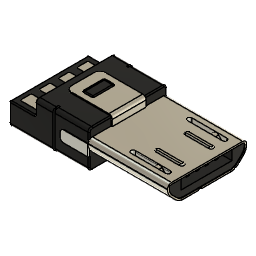
Micro-B (Autodesk Fusion 360 design; units mm, degrees)
Autodesk Fusion 360 part; units mm, degrees
sketch "Sketch1" plane through (0, 0, 0) normal (0, 0, 1) x (1, 0, 0)
  line L0 (3.35, 3.5) -> (-3.35, 3.5)
  line L1 (-3.35, 3.5) -> (-3.35, -3.5)
  line L2 (-3.35, -3.5) -> (3.35, -3.5)
  line L3 (3.35, -3.5) -> (3.35, 3.5)
  line L4 (3.35, 3.5) -> (-3.35, -3.5) construction
  line L5 (-3.35, 3.5) -> (3.35, -3.5) construction
  dimension "d1" = 6.7
  dimension "d2" = 7
  constraint horizontal L0
  constraint perpendicular L0 L1
  constraint parallel L0 L2
  constraint parallel L1 L3
  constraint coincident L4 origin
  constraint coincident L5 origin
  measures "d1" distance of L1.end L2.end
  measures "d2" distance of L0.end L1.end
extrude "Extrude1" add sketch "Sketch1" along normal blind 3.3
sketch "Sketch2" plane through (0, 0, 3.3) normal (0, 0, 1) x (-1, 0, 0)
  line L0 (-3.35, 3.5) -> (-3.35, -3.5)
  line L1 (-3.35, -3.5) -> (3.35, -3.5)
  line L2 (3.35, -3.5) -> (3.35, 3.5)
  line L3 (3.35, 3.5) -> (-3.35, 3.5)
  line L4 (3.35, -3.5) -> (1.35, -3.5)
  line L5 (1.35, -3.5) -> (1.35, 3.5)
  line L6 (1.35, 3.5) -> (3.35, 3.5)
  line L7 (3.35, 3.5) -> (3.35, -3.5)
  dimension "d5" = 2
  constraint horizontal L4
  constraint vertical L5
  constraint horizontal L6
  constraint vertical L7
  constraint coincident L3 L5.end
  constraint coincident L1.end L2.start
  measures "d5" distance of L1.end L4.end
extrude "Extrude2" cut sketch "Sketch2" against normal blind 1.3 contours L1 L2 L3 L4 L5 L6 L7
sketch "Sketch3" plane through (0, 0, 2) normal (0, 0, 1) x (-1, 0, 0)
  line L0 (3.35, 3.5) -> (1.35, 3.5)
  line L1 (1.35, 3.5) -> (1.35, -3.5)
  line L2 (1.35, -3.5) -> (3.35, -3.5)
  line L3 (3.35, -3.5) -> (3.35, 3.5)
  circle A0 centre (2.35, -2.5) radius 0.75
  line L4 (3.2, -3) -> (1.5, -3)
  line L5 (1.5, -3) -> (1.5, -2)
  line L6 (1.5, -2) -> (3.2, -2)
  line L7 (3.2, -2) -> (3.2, -3)
  line L8 (3.2, -3) -> (1.5, -2) construction
  line L9 (1.5, -3) -> (3.2, -2) construction
  line L10 (3.2, -0.35) -> (1.5, -0.35)
  line L11 (1.5, -0.35) -> (1.5, -1.35)
  line L12 (1.5, -1.35) -> (3.2, -1.35)
  line L13 (3.2, -1.35) -> (3.2, -0.35)
  line L14 (3.2, -0.35) -> (1.5, -1.35) construction
  line L15 (1.5, -0.35) -> (3.2, -1.35) construction
  point P0 (2.35, -2.5)
  point P1 (2.35, -0.85)
  dimension "d8" = 1.5
  dimension "d9" = 1
  dimension "d10" = 1
  dimension "d161" = 1.7
  dimension "d162" = 1
  dimension "d165" = 1.7
  dimension "d166" = 1
  dimension "d167" = 1.65
  dimension "d168" = 1
  constraint horizontal L4
  constraint perpendicular L4 L5
  constraint parallel L4 L6
  constraint parallel L5 L7
  constraint coincident L8 P0
  constraint coincident L9 P0
  constraint coincident P0 A0.centre
  constraint horizontal L10
  constraint perpendicular L10 L11
  constraint parallel L10 L12
  constraint parallel L11 L13
  constraint coincident L14 P1
  constraint coincident L15 P1
  measures "d8" diameter of A0
  measures "d9" distance of L2 P0
  measures "d10" distance of L1 P0
  measures "d161" distance of L5.end L6.end
  measures "d162" distance of L4.end L5.end
  measures "d165" distance of L11.end L12.end
  measures "d166" distance of L10.end L11.end
  measures "d167" distance of P0 P1
  measures "d168" distance of L3 P1
extrude "Extrude3" add sketch "Sketch3" along normal blind 0.001 contours A0 L4 L6 | A0 L4 L6 L7 | A0 L4 L5 L6
mirror "Mirror1" about plane through (0, 0, 0) normal (0, 1, 0) of "Extrude3"
sketch "Sketch4" plane through (0, 0, 0) normal (0, 0, -1) x (1, 0, 0)
  line L0 (3.35, -3.5) -> (3.35, 3.5)
  line L1 (3.35, 3.5) -> (-3.35, 3.5)
  line L2 (-3.35, 3.5) -> (-3.35, -3.5)
  line L3 (-3.35, -3.5) -> (3.35, -3.5)
  line L4 (-2.75, 2.75) -> (-1.95, 2.75)
  line L5 (-1.95, 2.75) -> (-1.95, -2.75)
  line L6 (-1.95, -2.75) -> (-2.75, -2.75)
  line L7 (-2.75, -2.75) -> (-2.75, 2.75)
  line L8 (-2.75, 2.75) -> (-1.95, -2.75) construction
  line L9 (-1.95, 2.75) -> (-2.75, -2.75) construction
  line L10 (0.35, -3.5) -> (0.2, -3.5)
  line L11 (0.2, -3.5) -> (0.2, 3.5)
  line L12 (0.2, 3.5) -> (0.35, 3.5)
  line L13 (0.35, 3.5) -> (0.35, -3.5)
  line L14 (3.35, -1.5) -> (-0.65, -1.5)
  line L15 (-0.65, -1.5) -> (-0.65, 1.5)
  line L16 (-0.65, 1.5) -> (3.35, 1.5)
  line L17 (3.35, 1.5) -> (3.35, -1.5)
  line L18 (3.35, -1.5) -> (3.45, -1.5)
  line L19 (3.45, -1.5) -> (3.45, 1.5)
  line L20 (3.45, 1.5) -> (3.35, 1.5)
  line L21 (3.35, 1.5) -> (3.35, -1.5)
  point P0 (-2.35, 0)
  dimension "d15" = 0.8
  dimension "d16" = 5.5
  dimension "d17" = 1
  dimension "d18" = 3.5
  dimension "d21" = 0.15
  dimension "d22" = 7
  dimension "d23" = 3
  dimension "d26" = 4
  dimension "d27" = 3
  dimension "d28" = 2
  dimension "d29" = 0.1
  dimension "d30" = 3
  constraint horizontal L4
  constraint perpendicular L4 L5
  constraint parallel L4 L6
  constraint parallel L5 L7
  constraint coincident L8 P0
  constraint coincident L9 P0
  constraint horizontal L10
  constraint vertical L11
  constraint horizontal L12
  constraint vertical L13
  constraint coincident L3 L10.start
  constraint horizontal L14
  constraint vertical L15
  constraint horizontal L16
  constraint vertical L17
  constraint coincident L0 L14.start
  constraint horizontal L18
  constraint vertical L19
  constraint horizontal L20
  constraint vertical L21
  measures "d15" distance of L5.end L6.end
  measures "d16" distance of L4.end L5.end
  measures "d17" distance of L2 P0
  measures "d18" distance of L3 P0
  measures "d21" distance of L10.start L10.end
  measures "d22" distance of L10.start L12.end
  measures "d23" distance of L0 L13
  measures "d26" distance of L14.start L14.end
  measures "d27" distance of L14.start L16.end
  measures "d28" distance of L3 L14
  measures "d29" distance of L14.start L18.end
  measures "d30" distance of L14.start L16.end
extrude "Extrude4" cut sketch "Sketch4" against normal blind 0.5 contours L4 L5 L6 L7
extrude "Extrude5" cut sketch "Sketch4" against normal blind 0.2 contours L3 L10 L11 L13 L14 | L11 L13 L14 L16 | L1 L11 L12 L13 L16
extrude "Extrude6" add sketch "Sketch4" along normal blind 0.1 contours L0 L13 L14 L16 L17 L21 | L0 L17 L18 L19 L20 L21 | L11 L13 L14 L16 | L11 L14 L15 L16
extrude "Extrude7" add 1 faces at (3.3833, -0.5, 0) along direction (0, 0, 1) blind 0.75
sketch "Sketch5" plane through (0, 0, -0.1) normal (0, 0, -1) x (1, 0, 0)
  line L0 (-0.65, -1.5) -> (3.45, -1.5)
  line L1 (3.45, -1.5) -> (3.45, 1.5)
  line L2 (3.45, 1.5) -> (-0.65, 1.5)
  line L3 (-0.65, 1.5) -> (-0.65, -1.5)
  line L4 (0.25, 1) -> (1.25, 1)
  line L5 (1.25, 1) -> (1.25, -1)
  line L6 (1.25, -1) -> (0.25, -1)
  line L7 (0.25, -1) -> (0.25, 1)
  line L8 (0.25, 1) -> (1.25, -1) construction
  line L9 (1.25, 1) -> (0.25, -1) construction
  point P0 (0.75, 0)
  dimension "d35" = 1
  dimension "d36" = 2
  dimension "d37" = 1.5
  dimension "d38" = 1.4
  constraint horizontal L4
  constraint perpendicular L4 L5
  constraint parallel L4 L6
  constraint parallel L5 L7
  constraint coincident L8 P0
  constraint coincident L9 P0
  measures "d35" distance of L5.end L6.end
  measures "d36" distance of L4.end L5.end
  measures "d37" distance of L0 P0
  measures "d38" distance of L3 P0
extrude "Extrude8" cut sketch "Sketch5" against normal blind 0.08 contours L4 L5 L6 L7
fillet "Fillet1" radius 0.5 2 edges at (-0.65, -1.5, -0.05) (-0.65, 1.5, -0.05)
fillet "Fillet1" radius 0.15 4 edges at (0.25, 1, -0.06) (1.25, 1, -0.06) (1.25, -1, -0.06) (0.25, -1, -0.06)
fillet "Fillet1" radius 0.3 1 edges at (3.45, 0, -0.1)
sketch "Sketch6" plane through (0, 0, -0.02) normal (0, 0, -1) x (1, 0, 0)
  arc A0 (0.4, 1) -> (0.25, 0.85) centre (0.4, 0.85) ccw
  line L0 (0.25, 0.85) -> (0.25, -0.85)
  arc A1 (0.25, -0.85) -> (0.4, -1) centre (0.4, -0.85) ccw
  line L1 (0.4, -1) -> (1.1, -1)
  arc A2 (1.1, -1) -> (1.25, -0.85) centre (1.1, -0.85) ccw
  line L2 (1.25, -0.85) -> (1.25, 0.85)
  arc A3 (1.25, 0.85) -> (1.1, 1) centre (1.1, 0.85) ccw
  line L3 (1.1, 1) -> (0.4, 1)
  line L4 (1.2, -0.85) -> (1.2, 0.85)
  arc A4 (1.2, 0.85) -> (1.1, 0.95) centre (1.1, 0.85) ccw
  line L5 (1.1, 0.95) -> (0.4, 0.95)
  arc A5 (0.4, 0.95) -> (0.3, 0.85) centre (0.4, 0.85) ccw
  line L6 (0.3, 0.85) -> (0.3, -0.85)
  arc A6 (0.3, -0.85) -> (0.4, -0.95) centre (0.4, -0.85) ccw
  line L7 (0.4, -0.95) -> (1.1, -0.95)
  arc A7 (1.1, -0.95) -> (1.2, -0.85) centre (1.1, -0.85) ccw
  dimension "d47" = -0.05
extrude "Extrude9" add sketch "Sketch6" along normal blind 0.1 contours L4 A4 L5 A5 L6 A6 L7 A7
fillet "Fillet2" radius 0.1 8 edges at (0.75, -0.95, -0.12) (0.3293, -0.9207, -0.12) (0.3, 0, -0.12) (0.3293, 0.9207, -0.12) (0.75, 0.95, -0.12) (1.1707, 0.9207, -0.12) (1.2, 0, -0.12) (1.1707, -0.9207, -0.12)
ref_plane "WorkPlane1" through (1.85, -2.5, 1.65) normal (0, 0, -1) x (-1, 0, 0)
mirror "Mirror2" about plane through (1.85, -2.5, 1.65) normal (0, 0, -1) of "Extrude6", "Extrude7", "Extrude8", "Fillet1", "Extrude9", "Fillet2"
sketch "Sketch7" plane through (0, -3.5, 0) normal (0, -1, 0) x (1, 0, 0)
  line L0 (0.2, 0) -> (0.2, 0.2)
  line L1 (0.2, 0.2) -> (0.35, 0.2)
  line L2 (0.35, 0.2) -> (0.35, 0)
  line L3 (0.35, 0) -> (3.35, 0)
  line L4 (3.35, 0) -> (3.35, 3.3)
  line L5 (3.35, 3.3) -> (-1.35, 3.3)
  line L6 (-1.35, 3.3) -> (-1.35, 2)
  line L7 (-1.35, 2) -> (-3.35, 2)
  line L8 (-3.35, 2) -> (-3.35, 0)
  line L9 (-3.35, 0) -> (0.2, 0)
  line L10 (0.35, 0.2) -> (0.2, 0.2)
  line L11 (0.2, 0.2) -> (0.2, 3.3)
  line L12 (0.2, 3.3) -> (0.35, 3.3)
  line L13 (0.35, 3.3) -> (0.35, 0.2)
  dimension "d54" = 0.15
  constraint horizontal L10
  constraint vertical L11
  constraint horizontal L12
  constraint vertical L13
  constraint coincident L5 L11.end
  constraint coincident L1.end L2.start
  measures "d54" distance of L1.end L0.end
extrude "Extrude10" cut sketch "Sketch7" against normal blind 0.2 contours L1 L5 L10 L11 L12 L13
mirror "Mirror3" about plane through (0, 0, 0) normal (0, 1, 0) of "Extrude10"
sketch "Sketch8" plane through (3.35, 0, 0) normal (1, 0, 0) x (0, 1, 0)
  line L0 (-1.5, 2.55) -> (-1.5, 3.3)
  line L1 (-1.5, 3.3) -> (-3.5, 3.3)
  line L2 (-3.5, 3.3) -> (-3.5, 0)
  line L3 (-3.5, 0) -> (-1.5, 0)
  line L4 (-1.5, 0) -> (-1.5, 0.75)
  line L5 (-1.5, 0.75) -> (1.5, 0.75)
  line L6 (1.5, 0.75) -> (1.5, 0)
  line L7 (1.5, 0) -> (3.5, 0)
  line L8 (3.5, 0) -> (3.5, 3.3)
  line L9 (3.5, 3.3) -> (1.5, 3.3)
  line L10 (1.5, 3.3) -> (1.5, 2.55)
  line L11 (1.5, 2.55) -> (-1.5, 2.55)
  line L12 (1.5, 2.55) -> (3.5, 2.55)
  line L13 (3.5, 2.55) -> (-3.5, 2.55)
  line L14 (-3.5, 2.55) -> (-3.5, 0.75)
  line L15 (-3.5, 0.75) -> (3.5, 0.75)
  line L16 (3.5, 0.75) -> (3.5, 2.55)
  dimension "d59" = 1.8
  constraint coincident L10.end L11.start
  constraint coincident L8 L12.end
  constraint perpendicular L8 L12
  constraint horizontal L13
  constraint vertical L14
  constraint horizontal L15
  constraint vertical L16
  constraint coincident L2 L14.end
  measures "d59" distance of L12.end L15.end
extrude "Extrude11" add sketch "Sketch8" along normal blind 7 contours L2 L5 L8 L11 L12 L13 L14 L15 L16
extrude "Extrude12" add 1 faces at (-3.35, 1.1667, 0.6667) along direction (-1, 0, 0) blind 0.3
sketch "Sketch9" plane through (0, -3.5, 0) normal (0, -1, 0) x (1, 0, 0)
  line L0 (0.35, 3.3) -> (0.35, 0)
  line L1 (0.35, 0) -> (3.35, 0)
  line L2 (3.35, 0) -> (3.35, 0.75)
  line L3 (3.35, 0.75) -> (10.35, 0.75)
  line L4 (10.35, 0.75) -> (10.35, 2.55)
  line L5 (10.35, 2.55) -> (3.35, 2.55)
  line L6 (3.35, 2.55) -> (3.35, 3.3)
  line L7 (3.35, 3.3) -> (0.35, 3.3)
  line L8 (3.35, 2.55) -> (3.35, 0.75)
  line L9 (3.35, 2.15) -> (0.85, 2.15)
  line L10 (0.85, 2.15) -> (0.85, 1.15)
  line L11 (0.85, 1.15) -> (3.35, 1.15)
  line L12 (3.35, 1.15) -> (3.35, 2.15)
  dimension "d64" = 2.5
  dimension "d65" = 1
  dimension "d66" = 1.15
  constraint coincident L5.end L6.start
  constraint coincident L2.end L3.start
  constraint horizontal L9
  constraint vertical L10
  constraint horizontal L11
  constraint vertical L12
  constraint coincident L8 L9.start
  measures "d64" distance of L9.start L9.end
  measures "d65" distance of L9.start L11.end
  measures "d66" distance of L7 L9
extrude "Extrude13" cut sketch "Sketch9" against normal blind 0.05 contours L0 L1 L2 L6 L7 L8 L9 L10 L11
fillet "Fillet3" radius 0.3 2 edges at (0.85, -3.475, 2.15) (0.85, -3.475, 1.15)
mirror "Mirror4" about plane through (0, 0, 0) normal (0, 1, 0) of "Extrude13", "Fillet3"
sketch "Sketch10" plane through (0, 0, 2.55) normal (0, 0, 1) x (-1, 0, 0)
  line L0 (-3.35, -1.5) -> (-3.45, -1.5)
  line L1 (-3.45, -1.5) -> (-3.45, 1.5)
  line L2 (-3.45, 1.5) -> (-3.35, 1.5)
  line L3 (-3.35, 1.5) -> (-3.35, 3.45)
  line L4 (-3.35, 3.45) -> (-3.35, 3.5)
  line L5 (-3.35, 3.5) -> (-10.35, 3.5)
  line L6 (-10.35, 3.5) -> (-10.35, -3.5)
  line L7 (-10.35, -3.5) -> (-3.35, -3.5)
  line L8 (-3.35, -3.5) -> (-3.35, -3.45)
  line L9 (-3.35, -3.45) -> (-3.35, -1.5)
  line L10 (-6.1, -2.3) -> (-9.6, -2.3)
  line L11 (-9.6, -2.3) -> (-9.6, -2.7)
  line L12 (-9.6, -2.7) -> (-6.1, -2.7)
  line L13 (-6.1, -2.7) -> (-6.1, -2.3)
  line L14 (-6.1, -2.3) -> (-9.6, -2.7) construction
  line L15 (-9.6, -2.3) -> (-6.1, -2.7) construction
  line L16 (-7.1, -1.1) -> (-9.6, -1.1)
  line L17 (-9.6, -1.1) -> (-9.6, -1.5)
  line L18 (-9.6, -1.5) -> (-7.1, -1.5)
  line L19 (-7.1, -1.5) -> (-7.1, -1.1)
  line L20 (-7.1, -1.1) -> (-9.6, -1.5) construction
  line L21 (-9.6, -1.1) -> (-7.1, -1.5) construction
  point P0 (-7.85, -2.5)
  point P1 (-8.35, -1.3)
  dimension "d73" = 0.4
  dimension "d74" = 3.5
  dimension "d75" = 2.5
  dimension "d76" = 1
  dimension "d77" = 2.5
  dimension "d78" = 0.4
  dimension "d79" = 1
  dimension "d80" = 2
  constraint horizontal L10
  constraint perpendicular L10 L11
  constraint parallel L10 L12
  constraint parallel L11 L13
  constraint coincident L14 P0
  constraint coincident L15 P0
  constraint horizontal L16
  constraint perpendicular L16 L17
  constraint parallel L16 L18
  constraint parallel L17 L19
  constraint coincident L20 P1
  constraint coincident L21 P1
  measures "d73" distance of L10.end L11.end
  measures "d74" distance of L11.end L12.end
  measures "d75" distance of L6 P0
  measures "d76" distance of L7 P0
  measures "d77" distance of L17.end L18.end
  measures "d78" distance of L16.end L17.end
  measures "d79" distance of L10 P1
  measures "d80" distance of L6 P1
extrude "Extrude14" cut sketch "Sketch10" against normal blind 0.5 contours L10 L11 L12 L13
extrude "Extrude15" add sketch "Sketch10" along normal blind 0.1 contours L16 L17 L18 L19
sketch "Sketch11" plane through (0, 0, 2.05) normal (0, 0, 1) x (-1, 0, 0)
  line L0 (-6.1, -2.7) -> (-6.1, -2.3)
  line L1 (-6.1, -2.3) -> (-9.6, -2.3)
  line L2 (-9.6, -2.3) -> (-9.6, -2.7)
  line L3 (-9.6, -2.7) -> (-6.1, -2.7)
  line L4 (-6.125, -2.325) -> (-9.575, -2.325)
  line L5 (-9.575, -2.325) -> (-9.575, -2.675)
  line L6 (-9.575, -2.675) -> (-6.125, -2.675)
  line L7 (-6.125, -2.675) -> (-6.125, -2.325)
  line L8 (-8.075, -2.675) -> (-9.075, -2.675)
  line L9 (-9.075, -2.675) -> (-9.075, -2.325)
  line L10 (-9.075, -2.325) -> (-8.075, -2.325)
  line L11 (-8.075, -2.325) -> (-8.075, -2.675)
  dimension "d85" = -0.025
  dimension "d86" = 1
  dimension "d87" = 0.5
  dimension "d88" = 0.35
  constraint horizontal L8
  constraint vertical L9
  constraint horizontal L10
  constraint vertical L11
  constraint coincident L6 L8.start
  measures "d86" distance of L8.start L8.end
  measures "d87" distance of L5 L9
  measures "d88" distance of L8.end L9.end
extrude "Extrude16" add sketch "Sketch11" along normal blind 0.5 contours L4 L6 L8 L9 L10 L11
chamfer "Chamfer1" distance 0.5 distance2 0.5 1 edges at (9.075, 2.5, 2.55) measured on face at (8.7417, 2.4417, 2.55)
chamfer "Chamfer1" distance 0.2 distance2 0.5 1 edges at (8.075, 2.5, 2.55) measured on face at (8.7417, 2.4417, 2.55)
fillet "Fillet4" radius 0.3 2 edges at (8.575, 2.5, 2.55) (8.275, 2.5, 2.55)
fillet "Fillet4" radius 0.2 8 edges at (9.6, 2.7, 2.3) (9.6, 2.3, 2.3) (6.1, 2.3, 2.3) (6.1, 2.7, 2.3) (7.1, 1.1, 2.6) (7.1, 1.5, 2.6) (9.6, 1.1, 2.6) (9.6, 1.5, 2.6)
fillet "Fillet5" radius 0.1 4 edges at (7.1, 1.3, 2.65) (8.35, 1.1, 2.65) (9.6, 1.3, 2.65) (8.35, 1.5, 2.65)
mirror "Mirror5" about plane through (0, 0, 0) normal (0, 1, 0) of "Extrude14", "Extrude15", "Extrude16", "Chamfer1", "Fillet4", "Fillet5"
sketch "Sketch12" plane through (0, 0, 0.75) normal (0, 0, -1) x (1, 0, 0)
  line L0 (3.45, -1.5) -> (3.35, -1.5)
  line L1 (3.35, -1.5) -> (3.35, -3.45)
  line L2 (3.35, -3.45) -> (3.35, -3.5)
  line L3 (3.35, -3.5) -> (10.35, -3.5)
  line L4 (10.35, -3.5) -> (10.35, 3.5)
  line L5 (10.35, 3.5) -> (3.35, 3.5)
  line L6 (3.35, 3.5) -> (3.35, 3.45)
  line L7 (3.35, 3.45) -> (3.35, 1.5)
  line L8 (3.35, 1.5) -> (3.45, 1.5)
  line L9 (3.45, 1.5) -> (3.45, -1.5)
  arc A0 (6.0406, -0.465) -> (6.3156, -0.74) centre (6.3156, -0.465) ccw
  arc A1 (6.2406, -0.465) -> (6.22, -0.3765) centre (6.0406, -0.465) ccw
  arc A2 (4.8906, -0.465) -> (5.1656, -0.74) centre (5.1656, -0.465) ccw
  line L10 (6.0406, -0.465) -> (6.0406, -0.515)
  arc A3 (5.7656, -0.24) -> (5.4906, -0.515) centre (5.7656, -0.515) ccw
  arc A4 (11.2406, -0.465) -> (11.22, -0.3765) centre (11.0406, -0.465) ccw
  arc A5 (10.2156, -0.74) -> (10.4906, -0.465) centre (10.2156, -0.465) ccw
  arc A6 (6.2406, -0.465) -> (6.3156, -0.54) centre (6.3156, -0.465) ccw
  arc A7 (10.3112, -0.3765) -> (10.2906, -0.465) centre (10.4906, -0.465) ccw
  arc A8 (5.2156, -0.54) -> (5.2906, -0.465) centre (5.2156, -0.465) ccw
  arc A9 (6.3656, -0.74) -> (6.6406, -0.465) centre (6.3656, -0.465) ccw
  line L11 (6.3656, -0.54) -> (6.3156, -0.54)
  arc A10 (5.0906, -0.465) -> (5.1656, -0.54) centre (5.1656, -0.465) ccw
  line L12 (5.1656, -0.54) -> (5.2156, -0.54)
  line L13 (6.3656, -0.74) -> (6.3156, -0.74)
  line L14 (11.3656, -0.74) -> (11.3156, -0.74)
  line L15 (6.3656, -0.74) -> (6.3156, -0.74)
  line L16 (5.4906, -0.465) -> (5.4906, -0.515)
  arc A11 (6.3656, -0.74) -> (6.6406, -0.465) centre (6.3656, -0.465) ccw
  arc A12 (11.2406, -0.465) -> (11.3156, -0.54) centre (11.3156, -0.465) ccw
  arc A13 (8.8656, -0.54) -> (8.9406, -0.465) centre (8.8656, -0.465) ccw
  line L17 (6.3656, -0.54) -> (6.3156, -0.54)
  line L18 (11.0406, -0.515) -> (11.0406, -0.465)
  arc A14 (6.3656, -0.54) -> (6.4406, -0.465) centre (6.3656, -0.465) ccw
  arc A15 (6.2406, -0.465) -> (6.3156, -0.54) centre (6.3156, -0.465) ccw
  line L19 (7.6656, -0.54) -> (7.7156, -0.54)
  arc A16 (11.0406, -0.465) -> (11.3156, -0.74) centre (11.3156, -0.465) ccw
  line L20 (10.4906, -0.515) -> (10.4906, -0.465)
  arc A17 (6.0406, -0.515) -> (5.7656, -0.24) centre (5.7656, -0.515) ccw
  arc A18 (11.3656, -0.74) -> (11.6406, -0.465) centre (11.3656, -0.465) ccw
  arc A19 (5.3112, -0.3765) -> (5.2906, -0.465) centre (5.4906, -0.465) ccw
  arc A20 (10.0906, -0.465) -> (10.1656, -0.54) centre (10.1656, -0.465) ccw
  arc A21 (5.2156, -0.74) -> (5.4906, -0.465) centre (5.2156, -0.465) ccw
  arc A22 (4.8906, -0.465) -> (5.1656, -0.74) centre (5.1656, -0.465) ccw
  arc A23 (11.0406, -0.515) -> (10.7656, -0.24) centre (10.7656, -0.515) ccw
  arc A24 (6.0406, -0.465) -> (6.3156, -0.74) centre (6.3156, -0.465) ccw
  arc A25 (9.8906, -0.465) -> (10.1656, -0.74) centre (10.1656, -0.465) ccw
  arc A26 (5.0906, -0.465) -> (5.1656, -0.54) centre (5.1656, -0.465) ccw
  arc A27 (6.0406, -0.515) -> (5.7656, -0.24) centre (5.7656, -0.515) ccw
  arc A28 (6.2406, -0.465) -> (6.22, -0.3765) centre (6.0406, -0.465) ccw
  arc A29 (5.3112, -0.3765) -> (5.2906, -0.465) centre (5.4906, -0.465) ccw
  arc A30 (5.2156, -0.74) -> (5.4906, -0.465) centre (5.2156, -0.465) ccw
  arc A31 (5.7656, -0.24) -> (5.4906, -0.515) centre (5.7656, -0.515) ccw
  arc A32 (5.2156, -0.54) -> (5.2906, -0.465) centre (5.2156, -0.465) ccw
  line L21 (3.7906, 3.8194) -> (3.7906, -2.5806)
  line L22 (12.1906, 3.8194) -> (3.7906, 3.8194)
  line L23 (3.7906, -2.5806) -> (12.1906, -2.5806)
  line L24 (8.5406, -0.465) -> (8.5406, -0.515)
  line L25 (9.1406, 0.51) -> (9.1406, -0.465)
  line L26 (10.0906, 0.51) -> (10.0906, -0.465)
  line L27 (11.4406, 0.51) -> (11.4406, -0.465)
  arc A33 (5.7656, -0.04) -> (5.3112, -0.3765) centre (5.7656, -0.515) ccw
  line L28 (9.8906, 0.51) -> (9.8906, -0.465)
  line L29 (11.1, -2.515) -> (11.1, 3.735)
  arc A34 (8.2656, -0.24) -> (7.9906, -0.515) centre (8.2656, -0.515) ccw
  line L30 (4.45, 0.61) -> (11.1, 0.61)
  line L31 (12.1906, -2.5806) -> (12.1906, 3.8194)
  line L32 (4.45, -2.515) -> (11.1, -2.515)
  line L33 (11.1, 0.61) -> (12.1906, 0.61)
  line L34 (11.1, 0.71) -> (12.1906, 0.71)
  line L35 (4.45, 0.71) -> (11.1, 0.71)
  circle A35 centre (9.1906, 2.6194) radius 0.3732
  line L36 (11.6406, 0.51) -> (12.1906, 0.51)
  line L37 (11.4406, 0.51) -> (11.4406, 0.71)
  line L38 (8.9406, 0.51) -> (8.9406, 0.71)
  arc A36 (7.7156, -0.54) -> (7.7906, -0.465) centre (7.7156, -0.465) ccw
  line L39 (5.0906, 0.51) -> (5.0906, 0.71)
  line L40 (6.6406, 0.51) -> (6.6406, -0.465)
  line L41 (5.0906, 0.51) -> (5.0906, -0.465)
  arc A37 (8.72, -0.3765) -> (8.2656, -0.04) centre (8.2656, -0.515) ccw
  line L42 (4.45, 0.51) -> (3.7906, 0.51)
  arc A38 (7.8112, -0.3765) -> (7.7906, -0.465) centre (7.9906, -0.465) ccw
  line L43 (4.45, 0.71) -> (3.7906, 0.71)
  line L44 (8.9406, 0.51) -> (8.9406, -0.465)
  line L45 (7.5906, 0.51) -> (7.5906, 0.71)
  line L46 (4.45, 0.51) -> (11.1, 0.51)
  line L47 (10.0906, 0.51) -> (10.0906, 0.71)
  line L48 (6.4406, 0.51) -> (6.4406, 0.71)
  line L49 (7.6656, -0.74) -> (7.7156, -0.74)
  line L50 (6.6406, 0.51) -> (6.6406, -0.465)
  arc A39 (6.22, -0.3765) -> (5.7656, -0.04) centre (5.7656, -0.515) ccw
  arc A40 (8.5406, -0.465) -> (8.8156, -0.74) centre (8.8156, -0.465) ccw
  line L51 (7.5906, 0.51) -> (7.5906, -0.465)
  line L52 (4.8906, 0.51) -> (4.8906, -0.465)
  arc A41 (8.7406, -0.465) -> (8.8156, -0.54) centre (8.8156, -0.465) ccw
  line L53 (4.45, 3.735) -> (4.45, -2.515)
  arc A42 (8.5406, -0.515) -> (8.2656, -0.24) centre (8.2656, -0.515) ccw
  line L54 (10.1656, -0.74) -> (10.2156, -0.74)
  arc A43 (8.8656, -0.74) -> (9.1406, -0.465) centre (8.8656, -0.465) ccw
  line L55 (11.3656, -0.54) -> (11.3156, -0.54)
  line L56 (5.1656, -0.74) -> (5.2156, -0.74)
  line L57 (6.4406, 0.51) -> (6.4406, -0.465)
  arc A44 (8.7406, -0.465) -> (8.72, -0.3765) centre (8.5406, -0.465) ccw
  line L58 (7.9906, -0.515) -> (7.9906, -0.465)
  arc A45 (7.5906, -0.465) -> (7.6656, -0.54) centre (7.6656, -0.465) ccw
  arc A46 (5.7656, -0.04) -> (5.3112, -0.3765) centre (5.7656, -0.515) ccw
  arc A47 (11.22, -0.3765) -> (10.7656, -0.04) centre (10.7656, -0.515) ccw
  arc A48 (10.7656, -0.04) -> (10.3112, -0.3765) centre (10.7656, -0.515) ccw
  arc A49 (10.2156, -0.54) -> (10.2906, -0.465) centre (10.2156, -0.465) ccw
  arc A50 (8.2656, -0.04) -> (7.8112, -0.3765) centre (8.2656, -0.515) ccw
  arc A51 (11.3656, -0.54) -> (11.4406, -0.465) centre (11.3656, -0.465) ccw
  arc A52 (7.7156, -0.74) -> (7.9906, -0.465) centre (7.7156, -0.465) ccw
  line L59 (7.3906, 0.51) -> (7.3906, -0.465)
  line L60 (8.8656, -0.54) -> (8.8156, -0.54)
  line L61 (11.6406, 0.51) -> (11.6406, -0.465)
  arc A53 (10.7656, -0.24) -> (10.4906, -0.515) centre (10.7656, -0.515) ccw
  line L62 (10.1656, -0.54) -> (10.2156, -0.54)
  line L63 (8.8656, -0.74) -> (8.8156, -0.74)
  arc A54 (7.3906, -0.465) -> (7.6656, -0.74) centre (7.6656, -0.465) ccw
  circle A55 centre (9.1906, -1.3806) radius 0.3732
  line L64 (3.7906, 0.71) -> (3.45, 0.71)
  line L65 (3.7906, 0.51) -> (3.45, 0.51)
  point P0 (6.6406, -0.74)
  point P1 (4.8906, -0.74)
  point P2 (6.0406, -0.74)
  point P3 (5.4906, -0.24)
  point P4 (6.0406, -0.24)
  point P5 (5.4906, -0.74)
  dimension "d103" = 0.2
  dimension "d104" = 0.1
  dimension "d105" = 0.1
  dimension "d106" = 1.25
  dimension "d107" = 1.25
  dimension "d108" = 0.6
  dimension "d109" = 1.75
  dimension "d110" = 0.6
  dimension "d111" = 0.5
  dimension "d112" = 0.5
  dimension "d113" = 0.275
  dimension "d114" = 0.275
  dimension "d115" = 0.275
  dimension "d116" = 0.275
  dimension "d117" = 1.75
  dimension "d118" = 0.275
  dimension "d119" = 0.275
  dimension "d120" = 1.75
  dimension "d121" = 0.275
  dimension "d122" = 0.275
  constraint midpoint L30.start L53
  constraint perpendicular L30 L53
  constraint coincident L42.start L53
  constraint coincident L46.end L29
  constraint perpendicular L29 L46
  constraint coincident L35.start L53
  constraint coincident L34.start L29
  constraint perpendicular L29 L35
  constraint coincident L40.start L46
  constraint perpendicular L46 L50
  constraint coincident L52.start L46
  constraint perpendicular L46 L52
  constraint perpendicular L13 L50
  constraint perpendicular L52 L56
  constraint perpendicular L10 L13
  constraint perpendicular L16 L56
  constraint coincident P0 L50
  constraint coincident P0 L13
  constraint tangent A9 L50
  constraint tangent A9 L13
  constraint coincident P2 L13
  constraint coincident P2 L10
  constraint tangent L13 A24
  constraint tangent L10 A24
  constraint equal A9 A24
  constraint coincident P5 L56
  constraint coincident P5 L16
  constraint tangent A30 L56
  constraint tangent L16 A30
  constraint equal A9 A30
  constraint coincident P1 L52
  constraint coincident P1 L56
  constraint tangent A22 L52
  constraint tangent A22 L56
  constraint equal A9 A22
  constraint coincident P4 L10
  constraint tangent L10 A27
  constraint coincident P3 L16
  constraint tangent A3 L16
  constraint equal A3 A27
  constraint coincident A3.start A17.end
  constraint coincident L39.end L35
  constraint perpendicular L35 L39
  constraint coincident L48.end L35
  constraint perpendicular L35 L48
  constraint perpendicular L15 L40
  constraint tangent A11 L40
  constraint tangent L15 A11
  constraint tangent A0 L15
  constraint equal A0 A11
  constraint equal A11 A21
  constraint equal A2 A11
  constraint equal A17 A31
  constraint perpendicular L49 L59
  constraint tangent L25 A43
  constraint tangent L49 A52
  constraint equal A43 A52
  constraint tangent A40 L63
  constraint perpendicular L28 L54
  constraint tangent A18 L61
  constraint tangent A5 L54
  constraint equal A5 A18
  constraint tangent L14 A16
  constraint coincident A43.start L63
  constraint tangent L24 A42
  constraint tangent L58 A52
  constraint coincident A4.centre L18.end
  constraint tangent L18 A16
  constraint coincident A5.end A7.centre
  constraint tangent A5 L20
  constraint coincident L45.end L35
  constraint perpendicular L35 L45
  constraint coincident L38.end L35
  constraint perpendicular L35 L38
  constraint coincident L47.end L35
  constraint perpendicular L35 L47
  constraint coincident L33.end L31
  constraint perpendicular L31 L33
  constraint coincident L36.end L31
  constraint perpendicular L31 L36
  constraint coincident L34.end L31
  constraint perpendicular L31 L34
  constraint coincident L37.end L34
  constraint perpendicular L34 L37
  constraint coincident L42.end L21
  constraint perpendicular L21 L42
  constraint coincident L43.end L21
  constraint perpendicular L21 L43
  constraint coincident L9 L64.end
  constraint perpendicular L9 L64
  constraint coincident L9 L65.end
  constraint perpendicular L9 L65
  measures "d104" distance of L30 L46
  measures "d105" distance of L30 L35
  measures "d106" distance of L40.start P0
  measures "d107" distance of P1 L52.start
  measures "d108" distance of P0 P2
  measures "d109" distance of L50 L52
  measures "d110" distance of P1 P5
  measures "d111" distance of P2 P4
  measures "d112" distance of P3 P5
  measures "d113" radius of A9
  measures "d114" radius of A27
  measures "d115" radius of A11
  measures "d116" radius of A17
  measures "d117" distance of L25 L59
  measures "d118" radius of A43
  measures "d119" radius of A42
  measures "d120" distance of L28 L61
  measures "d121" radius of A18
  measures "d122" radius of A23
extrude "Extrude17" cut sketch "Sketch12" against normal blind 0.1 contours L9 L21 L64 L65 | L21 L42 L43 L53 | L30 L39 L46 L53 | L30 L35 L39 L53 | A0 A1 A2 L10 A3 A6 A8 A9 L11 A10 L12 L13 L15 L16 A11 L17 A14 A15 A17 A19 A21 A22 A24 A26 A27 A28 A29 A30 A31 A32 A33 L40 L41 L46 L50 A39 L52 L56 L57 A46 | L30 L35 L45 L48 | L30 L45 L46 L48 | L4 L30 L35 L47 | L4 L30 L46 L47 | L30 L35 L38 L47 | A13 L19 L24 L25 A34 A36 A37 A38 L44 L46 L49 A40 L51 A41 A42 A43 A44 L58 A45 A50 A52 L59 L60 L63 A54 | L30 L38 L46 L47
fillet "Fillet6" radius 0.1 8 edges at (8.9406, -0.71, 0.8) (9.1406, -0.51, 0.8) (7.5906, -0.71, 0.8) (7.3906, -0.51, 0.8) (6.6406, -0.51, 0.8) (6.4406, -0.71, 0.8) (5.0906, -0.71, 0.8) (4.8906, -0.51, 0.8)
chamfer "Chamfer2" distance 1 distance2 1 2 edges at (6.85, -3.5, 0.75) (6.85, 3.5, 0.75) measured on face at (8.0167, -3.5, 1.8167) measured on face at (6.7016, 2.5791, 0.75)
fillet "Fillet7" radius 0.35 2 edges at (6.85, -3.5, 2.55) (6.85, 3.5, 2.55)
fillet "Fillet7" radius 1 4 edges at (6.85, -3.5, 1.75) (6.85, -2.5, 0.75) (6.85, 2.5, 0.75) (6.85, 3.5, 1.75)
sketch "Sketch13" plane through (10.35, 0, 0) normal (1, 0, 0) x (0, 1, 0)
  arc A0 (3.2071, 1.4571) -> (3.5, 2.1642) centre (2.5, 2.1642) ccw
  line L0 (3.5, 2.1642) -> (3.5, 2.2)
  arc A1 (3.5, 2.2) -> (3.15, 2.55) centre (3.15, 2.2) ccw
  line L1 (3.15, 2.55) -> (-3.15, 2.55)
  arc A2 (-3.15, 2.55) -> (-3.5, 2.2) centre (-3.15, 2.2) ccw
  line L2 (-3.5, 2.2) -> (-3.5, 2.1642)
  arc A3 (-3.5, 2.1642) -> (-3.2071, 1.4571) centre (-2.5, 2.1642) ccw
  line L3 (-3.2071, 1.4571) -> (-2.7929, 1.0429)
  arc A4 (-2.7929, 1.0429) -> (-2.0858, 0.75) centre (-2.0858, 1.75) ccw
  line L4 (-2.0858, 0.75) -> (-0.71, 0.75)
  line L5 (-0.71, 0.75) -> (-0.71, 0.85)
  line L6 (-0.71, 0.85) -> (-0.51, 0.85)
  line L7 (-0.51, 0.85) -> (-0.51, 0.75)
  line L8 (-0.51, 0.75) -> (2.0858, 0.75)
  arc A5 (2.0858, 0.75) -> (2.7929, 1.0429) centre (2.0858, 1.75) ccw
  line L9 (2.7929, 1.0429) -> (3.2071, 1.4571)
  line L10 (-0.71, 0.75) -> (-0.51, 0.75)
  line L11 (2.6868, 1.149) -> (3.101, 1.5632)
  arc A6 (3.101, 1.5632) -> (3.35, 2.1642) centre (2.5, 2.1642) ccw
  line L12 (3.35, 2.1642) -> (3.35, 2.2)
  arc A7 (3.35, 2.2) -> (3.15, 2.4) centre (3.15, 2.2) ccw
  line L13 (3.15, 2.4) -> (-3.15, 2.4)
  arc A8 (-3.15, 2.4) -> (-3.35, 2.2) centre (-3.15, 2.2) ccw
  line L14 (-3.35, 2.2) -> (-3.35, 2.1642)
  arc A9 (-3.35, 2.1642) -> (-3.101, 1.5632) centre (-2.5, 2.1642) ccw
  line L15 (-3.101, 1.5632) -> (-2.6868, 1.149)
  arc A10 (-2.6868, 1.149) -> (-2.0858, 0.9) centre (-2.0858, 1.75) ccw
  line L16 (-2.0858, 0.9) -> (-0.86, 0.9)
  line L17 (-0.86, 0.9) -> (-0.86, 1)
  line L18 (-0.86, 1) -> (-0.36, 1)
  line L19 (-0.36, 1) -> (-0.36, 0.9)
  line L20 (-0.36, 0.9) -> (2.0858, 0.9)
  arc A11 (2.0858, 0.9) -> (2.6868, 1.149) centre (2.0858, 1.75) ccw
  line L21 (-0.86, 0.9) -> (-0.36, 0.9)
  dimension "d133" = -0.15
  constraint coincident L4.end L5.start
  constraint coincident L7.end L8.start
extrude "Extrude18" cut sketch "Sketch13" against normal blind 0.05 contours L11 A6 L12 A7 L13 A8 L14 A9 L15 A10 L16 L17 L18 L19 L20 A11 | L17 L18 L19 L21
sketch "Sketch14" plane through (10.3, 0, 0) normal (1, 0, 0) x (0, 1, 0)
  line L0 (-2.0858, 0.9) -> (2.0858, 0.9)
  arc A0 (2.0858, 0.9) -> (2.6868, 1.149) centre (2.0858, 1.75) ccw
  line L1 (2.6868, 1.149) -> (3.101, 1.5632)
  arc A1 (3.101, 1.5632) -> (3.35, 2.1642) centre (2.5, 2.1642) ccw
  line L2 (3.35, 2.1642) -> (3.35, 2.2)
  arc A2 (3.35, 2.2) -> (3.15, 2.4) centre (3.15, 2.2) ccw
  line L3 (3.15, 2.4) -> (-3.15, 2.4)
  arc A3 (-3.15, 2.4) -> (-3.35, 2.2) centre (-3.15, 2.2) ccw
  line L4 (-3.35, 2.2) -> (-3.35, 2.1642)
  arc A4 (-3.35, 2.1642) -> (-3.101, 1.5632) centre (-2.5, 2.1642) ccw
  line L5 (-3.101, 1.5632) -> (-2.6868, 1.149)
  arc A5 (-2.6868, 1.149) -> (-2.0858, 0.9) centre (-2.0858, 1.75) ccw
  line L6 (-2.25, 2.4) -> (2.25, 2.4)
  line L7 (2.25, 2.4) -> (2.25, 1.5)
  line L8 (2.25, 1.5) -> (-2.25, 1.5)
  line L9 (-2.25, 1.5) -> (-2.25, 2.4)
  dimension "d136" = 4.5
  dimension "d137" = 0.9
  dimension "d138" = 1.1
  constraint horizontal L6
  constraint vertical L7
  constraint horizontal L8
  constraint vertical L9
  constraint coincident L3 L6.start
  measures "d136" distance of L6.start L6.end
  measures "d137" distance of L6.start L8.end
  measures "d138" distance of A3.end L9
extrude "Extrude19" cut sketch "Sketch14" against normal blind 5 contours L3 L6 L7 L8 L9
sketch "Sketch15" plane through (0, 0, 1.5) normal (0, 0, 1) x (-1, 0, 0)
  line L0 (-10.3, 2.25) -> (-10.3, -2.25)
  line L1 (-10.3, -2.25) -> (-5.3, -2.25)
  line L2 (-5.3, -2.25) -> (-5.3, 2.25)
  line L3 (-5.3, 2.25) -> (-10.3, 2.25)
  line L4 (-9.55, 1.6) -> (-8.05, 1.6)
  line L5 (-8.05, 1.6) -> (-8.05, 1.9)
  line L6 (-8.05, 1.9) -> (-9.55, 1.9)
  line L7 (-9.55, 1.9) -> (-9.55, 1.6)
  line L8 (-9.55, 1.6) -> (-8.05, 1.9) construction
  line L9 (-8.05, 1.6) -> (-9.55, 1.9) construction
  point P0 (-8.8, 1.75)
  dimension "d141" = 0.3
  dimension "d142" = 1.5
  dimension "d143" = 0.5
  dimension "d144" = 1.5
  constraint horizontal L4
  constraint perpendicular L4 L5
  constraint parallel L4 L6
  constraint parallel L5 L7
  constraint coincident L8 P0
  constraint coincident L9 P0
  measures "d141" distance of L4.end L5.end
  measures "d142" distance of L5.end L6.end
  measures "d143" distance of L3 P0
  measures "d144" distance of L0 P0
extrude "Extrude20" add sketch "Sketch15" along normal blind 0.4 contours L4 L5 L6 L7
fillet "Fillet8" radius 0.4 1 edges at (9.55, -1.75, 1.9)
fillet "Fillet8" radius 0.2 1 edges at (8.05, -1.75, 1.9)
pattern_linear "R-Pattern1" count 5 spacing 0.85 along (0, 1, 0) of "Extrude20", "Fillet8"
fillet "Fillet9" radius 0.3 10 edges at (1.85, -3.45, 3.3) (-0.575, -3.5, 3.3) (1.85, 3.45, 3.3) (-0.575, 3.5, 3.3) (1.85, -3.45, 0) (-1.725, -3.5, 0) (1.85, 3.45, 0) (-1.725, 3.5, 0) (0.275, -3.3, 3.3) (0.275, 3.3, 3.3)
fillet "Fillet10" radius 0.1 16 edges at (-2.5, -3.5, 2) (-2.5, 3.5, 2) (3.35, 3.45, 2.6901) (3.35, 3.3621, 3.2121) (3.35, 2.325, 3.3) (3.35, 2.325, 0) (3.35, 3.3621, 0.0879) (3.35, 3.45, 0.725) (3.35, 3.5, 1.65) (3.35, -3.45, 0.725) (3.35, -3.3621, 0.0879) (3.35, -2.325, 0) (3.35, -3.45, 2.6901) (3.35, -3.3621, 3.2121) (3.35, -2.325, 3.3) (3.35, -3.5, 1.65) 2 faces at (-3.65, -1.0667, 1.3333) (-1.35, -1.0667, 2.4333)
fillet "Fillet11" radius 0.1 4 edges at (-1.95, 2.75, 0.25) (-2.75, 2.75, 0.25) (-1.95, -2.75, 0.25) (-2.75, -2.75, 0.25) 1 faces at (-2.4833, 0.9167, 0.5)
fillet "Fillet12" radius 0.1 8 edges at (-3.2, 3, 2.0005) (-3.2, 2, 2.0005) (-1.5, 3, 2.0005) (-1.5, 2, 2.0005) (-3.2, -3, 2.0005) (-1.5, -3, 2.0005) (-3.2, -2, 2.0005) (-1.5, -2, 2.0005)
extrude "Extrude21" add sketch "Sketch3" along normal blind 0.001 contours L10 L11 L12 L13
fillet "Fillet13" radius 0.1 4 edges at (-3.2, 1.35, 2.0005) (-3.2, 0.35, 2.0005) (-1.5, 0.35, 2.0005) (-1.5, 1.35, 2.0005)
mirror "Mirror6" about plane through (0, 0, 0) normal (0, 1, 0) of "Extrude21", "Fillet13"
named bodies: "Micro-B"
